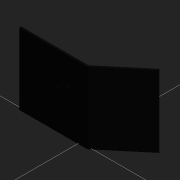
# Autodesk Inventor part: The Law Head
Saved by Autodesk Inventor 2015 SP1 (Build 190203100, 203)
## iProperties
Created: 2015-04-11
Part Number: The Law Head
Material: Aluminum 6061
Document SubType Name: Sheet Metal
Designer: datenney
Density: 2.7 g/cm^3
Sheet Metal Rule: Default
Appearance: Smooth - Black
Author: datenney
Autodesk Inventor part; units mm, degrees
ref_plane "YZ Plane" through (0, 0, 0) normal (1, 0, 0) x (0, 1, 0)
ref_plane "XZ Plane" through (0, 0, 0) normal (0, 1, 0) x (-1, 0, 0)
ref_plane "XY Plane" through (0, 0, 0) normal (0, 0, 1) x (1, 0, 0)
sketch "Sketch1" plane through (0, 0, 0) normal (0, 0, 1) x (1, 0, 0)
  line L0 (-88.9, -53.9686) -> (88.9, -53.9686)
  line L1 (88.9, -53.9686) -> (88.9, 53.9686)
  line L2 (88.9, 53.9686) -> (-88.9, 53.9686)
  line L3 (-88.9, 53.9686) -> (-88.9, -53.9686)
  line L4 (-88.9, -53.9686) -> (88.9, 53.9686) construction
  line L5 (88.9, -53.9686) -> (-88.9, 53.9686) construction
  line L6 (12.7, -53.9686) -> (12.7, 53.9686)
  point P0 (0, 0)
  dimension "d0" = 177.8
  dimension "d1" = 107.9373
  dimension "d2" = 76.2
  constraints: 14 end point, 2 midpoint, 2 parallel, 2 point on line, 1 horizontal, 1 perpendicular, 1 vertical
  measures "d0" distance of L2.end L1.end
  measures "d1" distance of L1.end L0.end
  measures "d2" distance between parallel lines of L1 L6
extrude "Plate1" add sketch "Sketch1" along normal blind 3.048
fold "Fold1" angle 40 bend radius 3.048 thickness 3.048 k factor 0.44 line from (12.7, -53.9686, 0) to (12.7, 53.9686, 0) line at bend centre moving side (1, 0, 0) folds toward (0, 0, -1)
sketch "Sketch2" plane through (0, 0, 0) normal (0, 0, -1) x (-1, 0, 0)
  circle A0 centre (195.2719, -111.7265) radius 2.4892 construction
  arc A1 (213.1717, -114.9789) -> (212.4185, -112.2526) centre (211.432, -113.9923) ccw construction
  line L0 (212.4185, -112.2526) -> (-7.8142, 12.628) construction
  arc A2 (-7.8142, 12.628) -> (-10.5405, 11.8747) centre (-8.8007, 10.8882) ccw projected
  line L1 (-10.5405, 11.8747) -> (-16.4595, 1.4361) projected
  arc A3 (-16.4595, 1.4361) -> (-15.7063, -1.2901) centre (-14.7198, 0.4496) ccw projected
  line L2 (204.5264, -126.1707) -> (-15.7063, -1.2901) construction
  arc A4 (204.5264, -126.1707) -> (207.2526, -125.4175) centre (205.5129, -124.4309) ccw construction
  line L3 (213.1717, -114.9789) -> (207.2526, -125.4175) construction
  circle A5 centre (202.231, -115.6725) radius 1.85 construction
  circle A6 centre (188.3129, -107.7804) radius 1.85 construction
  circle A7 centre (174.3948, -99.8883) radius 1.85 construction
  circle A8 centre (160.4766, -91.9961) radius 1.85 construction
  circle A9 centre (146.5585, -84.104) radius 1.85 construction
  circle A10 centre (132.6404, -76.2119) radius 1.85 construction
  circle A11 centre (118.7222, -68.3198) radius 1.85 construction
  circle A12 centre (104.8041, -60.4276) radius 1.85 construction
  circle A13 centre (90.886, -52.5355) radius 1.85 construction
  circle A14 centre (76.9678, -44.6434) radius 1.85 construction
  circle A15 centre (63.0497, -36.7513) radius 1.85 projected
  circle A16 centre (49.1316, -28.8591) radius 1.85 projected
  circle A17 centre (35.2135, -20.967) radius 1.85 projected
  circle A18 centre (21.2953, -13.0749) radius 1.85 projected
  circle A19 centre (7.3772, -5.1827) radius 1.85 projected
  circle A20 centre (-6.5409, 2.7094) radius 1.85 projected
  line L4 (-11.1679, 53.9686) -> (-11.1679, -53.9686) projected
  line L5 (88.9, -53.9686) -> (-11.1679, -53.9686) projected
  line L6 (88.9, 53.9686) -> (88.9, -53.9686) projected
  line L7 (-11.1679, 53.9686) -> (88.9, 53.9686) projected
  line L8 (0, 0) -> (-16.4595, 1.4361) construction
  line L9 (-16.4595, 1.4361) -> (-10.5405, 11.8747)
  line L10 (-7.8142, 12.628) -> (88.9, -42.2127)
  line L11 (88.9, -42.2127) -> (88.9, -60.606)
  line L12 (88.9, -53.9686) -> (88.9, 53.9686) projected
  line L13 (88.9, -60.606) -> (-15.7063, -1.2901)
  arc A21 (-16.4595, 1.4361) -> (-15.7063, -1.2901) centre (-14.7198, 0.4496) ccw
  arc A22 (-7.8142, 12.628) -> (-10.5405, 11.8747) centre (-8.8007, 10.8882) ccw
  line L14 (88.9, -60.606) -> (88.9, -53.9686)
  line L15 (88.9, -53.9686) -> (-11.1679, -53.9686)
  line L16 (-11.1679, -53.9686) -> (-11.1679, 53.9686)
  line L17 (-11.1679, 53.9686) -> (88.9, 53.9686)
  line L18 (88.9, 53.9686) -> (88.9, -53.9686)
  line L19 (-11.1679, 53.9686) -> (-70.3261, 53.9686)
  line L20 (-70.3261, 53.9686) -> (-70.3261, -53.9686)
  line L21 (-70.3261, -53.9686) -> (-11.1679, -53.9686)
  point P0 (-9.5539, 13.6145)
  dimension "d10" = 3.7
  dimension "d11" = 2
  constraints: 26 end point, 7 point on line, 6 tangent, 4 horizontal, 4 point on circle, 4 vertical, 2 centre point, 1 parallel
  measures "d10" diameter of A20
  measures "d11" radius of A22
hole "Hole1" at (70.3261, 53.9686, 0) at (70.3261, -53.9686, 0) at (6.5409, 2.7094, 0) at (-7.3772, -5.1827, 0) direction (0, 0, 1) diameter 3.7084 end through all
equation "\"d1\" = 1.4165 * d2"
equation "\"d2\" = 0.428571 * d0"
equation "\"d4\" = BendReliefWidth"
equation "\"d5\" = BendReliefDepth"
equation "\"d6\" = MinimumRemnant"
equation "\"d7\" = BendRadius"
equation "\"d9\" = BendRadius"
equation "\"d17\" = Thickness"
equation "\"BendRadius\" = Thickness"
equation "\"BendReliefWidth\" = Thickness"
equation "\"BendReliefDepth\" = 0.5 * Thickness"
equation "\"CornerReliefSize\" = 4 * Thickness"
equation "\"MinimumRemnant\" = 2 * Thickness"
equation "\"TransitionRadius\" = BendRadius"
equation "\"JacobiRadiusSize\" = BendRadius"
equation "\"GapSize\" = Thickness"
equation "\"d3\" = BendRadius"
equation "\"Thickness\" = 3.048"
body "Solid1"
